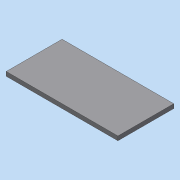
# Autodesk Inventor part: Camera-Holder_Side
Saved by Autodesk Inventor 2016 SP1 (Build 200210100, 210)
## iProperties
Created: 2016-02-07
Part Number: Camera-Holder_Side
Material: Generic
Document SubType Name: Modeling
Designer: Mohamed A.
Density: 1 g/cm^3
Appearance: Default
Author: Mohamed A.
Autodesk Inventor part; units mm, degrees
ref_plane "YZ Plane" through (0, 0, 0) normal (1, 0, 0) x (0, 1, 0)
ref_plane "XZ Plane" through (0, 0, 0) normal (0, 1, 0) x (-1, 0, 0)
ref_plane "XY Plane" through (0, 0, 0) normal (0, 0, 1) x (1, 0, 0)
sketch "Sketch1" plane through (0, 0, 0) normal (0, 0, 1) x (1, 0, 0)
  line L0 (-40, 20) -> (40, 20)
  line L1 (40, 20) -> (40, -20)
  line L2 (40, -20) -> (-40, -20)
  line L3 (-40, -20) -> (-40, 20)
  line L4 (-40, 20) -> (40, -20) construction
  line L5 (40, 20) -> (-40, -20) construction
  point P0 (0, 0)
  dimension "d0" = 80
  dimension "d1" = 40
  constraints: 12 end point, 2 midpoint, 2 parallel, 1 horizontal, 1 perpendicular
  measures "d0" distance of L1.end L2.end
  measures "d1" distance of L0.end L1.end
extrude "Extrusion1" add sketch "Sketch1" along normal mid plane 3
sketch "Sketch3" plane through (0, 0, 1.5) normal (0, 0, 1) x (1, 0, 0)
  line L0 (15.0052, -8) -> (12.0052, -8)
  line L1 (12.0052, -8) -> (12.0052, 8)
  line L2 (12.0052, 8) -> (15.0052, 8)
  line L3 (15.0052, 8) -> (15.0052, -8)
  line L4 (1.5, 8) -> (1.5, -8)
  line L5 (1.5, -8) -> (-1.5, -8)
  line L6 (-1.5, -8) -> (-1.5, 8)
  line L7 (-1.5, 8) -> (1.5, 8)
  line L8 (-11.9948, -8) -> (-14.9948, -8)
  line L9 (-14.9948, -8) -> (-14.9948, 8)
  line L10 (-14.9948, 8) -> (-11.9948, 8)
  line L11 (-11.9948, 8) -> (-11.9948, -8)
  line L12 (-40, -20) -> (40, -20) projected
  line L13 (40, 20) -> (-40, 20) projected
  line L14 (-40, 8.65) -> (-37, 8.65)
  line L15 (-37, 8.65) -> (-37, 7.5)
  line L16 (-37, 3.35) -> (-40, 3.35)
  line L17 (-40, 3.35) -> (-40, 8.65)
  line L18 (-40, 20) -> (-40, -20) projected
  line L19 (-40, 6) -> (-28.4075, 6) construction
  line L20 (-37, 7.5) -> (-35, 7.5)
  line L21 (-35, 7.5) -> (-35, 8.65)
  line L22 (-35, 8.65) -> (-32.6, 8.65)
  line L23 (-32.6, 8.65) -> (-32.6, 7.5)
  line L24 (-32.6, 7.5) -> (-32, 7.5)
  line L25 (-32, 7.5) -> (-32, 4.5)
  line L26 (-32, 4.5) -> (-32.6, 4.5)
  line L27 (-32.6, 4.5) -> (-32.6, 3.35)
  line L28 (-32.6, 3.35) -> (-35, 3.35)
  line L29 (-35, 3.35) -> (-35, 4.5)
  line L30 (-37, 4.5) -> (-35, 4.5)
  line L31 (-37, 4.5) -> (-37, 3.35)
  line L32 (-27.3167, 15) -> (-27.3167, 12)
  line L33 (-27.3167, 12) -> (-37, 12)
  line L34 (-37, 12) -> (-37, 15)
  line L35 (-37, 15) -> (-27.3167, 15)
  line L36 (-22.0167, 12) -> (-22.0167, 15)
  line L37 (-22.0167, 15) -> (-14.9948, 15)
  line L38 (-14.9948, 15) -> (-14.9948, 12)
  line L39 (-14.9948, 12) -> (-22.0167, 12)
  line L40 (27.3167, 12) -> (27.3167, 15)
  line L41 (27.3167, 15) -> (37, 15)
  line L42 (37, 15) -> (37, 12)
  line L43 (37, 12) -> (27.3167, 12)
  line L44 (22.0167, 15) -> (22.0167, 12)
  line L45 (22.0167, 12) -> (12.3333, 12)
  line L46 (12.3333, 12) -> (12.3333, 15)
  line L47 (12.3333, 15) -> (22.0167, 15)
  line L48 (27.3167, -15) -> (27.3167, -12)
  line L49 (27.3167, -12) -> (37, -12)
  line L50 (37, -12) -> (37, -15)
  line L51 (37, -15) -> (27.3167, -15)
  line L52 (22.0167, -12) -> (22.0167, -15)
  line L53 (22.0167, -15) -> (14.9948, -15)
  line L54 (14.9948, -15) -> (14.9948, -12)
  line L55 (14.9948, -12) -> (22.0167, -12)
  line L56 (-27.3167, -12) -> (-27.3167, -15)
  line L57 (-27.3167, -15) -> (-37, -15)
  line L58 (-37, -15) -> (-37, -12)
  line L59 (-37, -12) -> (-27.3167, -12)
  line L60 (-22.0167, -15) -> (-22.0167, -12)
  line L61 (-22.0167, -12) -> (-12.3333, -12)
  line L62 (-12.3333, -12) -> (-12.3333, -15)
  line L63 (-12.3333, -15) -> (-22.0167, -15)
  line L64 (-40, 20) -> (-37, 20)
  line L65 (-37, 20) -> (-37, 16.6667)
  line L66 (-37, 16.6667) -> (-40, 16.6667)
  line L67 (-40, 16.6667) -> (-40, 20)
  line L68 (-56.6135, 0) -> (53.1995, 0) construction
  line L69 (0, 37.0624) -> (0, -26.1921) construction
  line L70 (-40, -8.65) -> (-37, -8.65)
  line L71 (-37, -8.65) -> (-37, -7.5)
  line L72 (-37, -3.35) -> (-40, -3.35)
  line L73 (-40, -3.35) -> (-40, -8.65)
  line L74 (-37, -7.5) -> (-35, -7.5)
  line L75 (-35, -7.5) -> (-35, -8.65)
  line L76 (-35, -8.65) -> (-32.6, -8.65)
  line L77 (-32.6, -8.65) -> (-32.6, -7.5)
  line L78 (-32.6, -7.5) -> (-32, -7.5)
  line L79 (-32, -7.5) -> (-32, -4.5)
  line L80 (-32, -4.5) -> (-32.6, -4.5)
  line L81 (-32.6, -4.5) -> (-32.6, -3.35)
  line L82 (-32.6, -3.35) -> (-35, -3.35)
  line L83 (-35, -3.35) -> (-35, -4.5)
  line L84 (-37, -4.5) -> (-35, -4.5)
  line L85 (-37, -4.5) -> (-37, -3.35)
  line L86 (-40, -20) -> (-37, -20)
  line L87 (-37, -20) -> (-37, -16.6667)
  line L88 (-37, -16.6667) -> (-40, -16.6667)
  line L89 (-40, -16.6667) -> (-40, -20)
  line L90 (40, 8.65) -> (37, 8.65)
  line L91 (37, 8.65) -> (37, 7.5)
  line L92 (37, 3.35) -> (40, 3.35)
  line L93 (40, 3.35) -> (40, 8.65)
  line L94 (37, 7.5) -> (35, 7.5)
  line L95 (35, 7.5) -> (35, 8.65)
  line L96 (35, 8.65) -> (32.6, 8.65)
  line L97 (32.6, 8.65) -> (32.6, 7.5)
  line L98 (32.6, 7.5) -> (32, 7.5)
  line L99 (32, 7.5) -> (32, 4.5)
  line L100 (32, 4.5) -> (32.6, 4.5)
  line L101 (32.6, 4.5) -> (32.6, 3.35)
  line L102 (32.6, 3.35) -> (35, 3.35)
  line L103 (35, 3.35) -> (35, 4.5)
  line L104 (37, 4.5) -> (35, 4.5)
  line L105 (37, 4.5) -> (37, 3.35)
  line L106 (40, 20) -> (37, 20)
  line L107 (37, 20) -> (37, 16.6667)
  line L108 (37, 16.6667) -> (40, 16.6667)
  line L109 (40, 16.6667) -> (40, 20)
  line L110 (40, -20) -> (37, -20)
  line L111 (37, -20) -> (37, -16.6667)
  line L112 (37, -16.6667) -> (40, -16.6667)
  line L113 (40, -16.6667) -> (40, -20)
  line L114 (40, -8.65) -> (37, -8.65)
  line L115 (37, -8.65) -> (37, -7.5)
  line L116 (37, -7.5) -> (35, -7.5)
  line L117 (35, -7.5) -> (35, -8.65)
  line L118 (35, -8.65) -> (32.6, -8.65)
  line L119 (32.6, -8.65) -> (32.6, -7.5)
  line L120 (32.6, -7.5) -> (32, -7.5)
  line L121 (32, -7.5) -> (32, -4.5)
  line L122 (32, -4.5) -> (32.6, -4.5)
  line L123 (32.6, -4.5) -> (32.6, -3.35)
  line L124 (32.6, -3.35) -> (35, -3.35)
  line L125 (35, -3.35) -> (35, -4.5)
  line L126 (37, -4.5) -> (35, -4.5)
  line L127 (37, -4.5) -> (37, -3.35)
  line L128 (37, -3.35) -> (40, -3.35)
  line L129 (40, -3.35) -> (40, -8.65)
  line L130 (-24.6667, 17.1569) -> (-24.6667, 10.3686) construction
  circle A0 centre (-24.6667, 13.5) radius 1.4
  circle A1 centre (-24.6667, -13.5) radius 1.4
  circle A2 centre (24.6667, 13.5) radius 1.4
  circle A3 centre (24.6667, -13.5) radius 1.4
  point P0 (0, 0)
  dimension "d5" = 40
  dimension "d6" = 3
  dimension "d9" = 3
  dimension "d10" = 8
  dimension "d11" = 5
  dimension "d12" = 2.4
  dimension "d13" = 5.3
  dimension "d14" = 5
  dimension "d16" = 1.6667
  dimension "d17" = 12
  dimension "d18" = 6
  dimension "d21" = 5.3
  dimension "d22" = 2.65
  dimension "d23" = 2.8
  constraints: 256 end point, 60 symmetric about line, 38 point on line, 27 horizontal, 25 vertical, 11 perpendicular, 6 parallel, 4 centre point, 3 collinear, 50 other
  measures "d5" distance between parallel lines of L12 L13
  measures "d6" distance of L16.start L16.end
  measures "d9" distance between parallel lines of L26 L24
  measures "d10" distance between parallel lines of L18 L25
  measures "d11" distance between parallel lines of L18 L21
  measures "d12" distance between parallel lines of L21 L23
  measures "d13" distance between parallel lines of L28 L22
  measures "d14" distance between parallel lines of L13 L35
  measures "d16" distance between parallel lines of L35 L66
  measures "d17" distance from line of point (0, 0) L33
  measures "d18" distance between parallel lines of L33 L19
  measures "d21" distance between parallel lines of L32 L36
  measures "d22" distance between parallel lines of L130 L36
  measures "d23" diameter of A0
extrude "Extrusion2" cut sketch "Sketch3" against normal blind 3
equation "\"d16\" = 0.333333 * d14"
equation "\"d18\" = 0.5 * d17"
equation "\"d22\" = 0.5 * d21"
body "Solid1"
